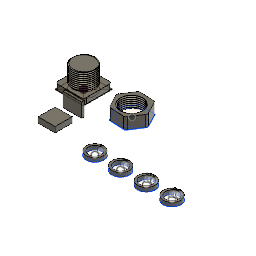
FineABSThreadTest (Autodesk Fusion 360 design; units mm, degrees)
Autodesk Fusion 360 part; units mm, degrees
sketch "Sketch1" plane through (0, 0, 0) normal (0, 1, 0) x (1, 0, 0)
  line L0 (25, 25) -> (-25, 25)
  line L1 (-25, 25) -> (-25, -25)
  line L2 (-25, -25) -> (25, -25)
  line L3 (25, -25) -> (25, 25)
  line L4 (25, 25) -> (-25, -25) construction
  line L5 (-25, 25) -> (25, -25) construction
  circle A0 centre (0, 0) radius 20
  circle A1 centre (85, 0) radius 20
  line L6 (100.5694, 24.4662) -> (71.5964, 25.7166)
  line L7 (71.5964, 25.7166) -> (56.027, 1.2504)
  line L8 (56.027, 1.2504) -> (69.4306, -24.4662)
  line L9 (69.4306, -24.4662) -> (98.4036, -25.7166)
  line L10 (98.4036, -25.7166) -> (113.973, -1.2504)
  line L11 (113.973, -1.2504) -> (100.5694, 24.4662)
  dimension "d1" = 50
  dimension "d2" = 50
  dimension "d3" = 40
  dimension "d4" = 40
  dimension "d5" = 29
  measures "d3" diameter of A0
  measures "d4" diameter of A1
extrude "Extrude1" add sketch "Sketch1" along normal blind 20 contours L6 L7 L8 L9 L10 L11 makes body 1
extrude "Extrude2" add sketch "Sketch1" along normal blind 10 separate body contours L0 L1 L2 L3 | A0 makes body 2
extrude "Extrude3" add sketch "Sketch1" along normal blind 40 contours A0 bodies 2
thread "Thread1" "ISO Metric profile 40.0 M40x3 6g" major diameter 39.7645 minor diameter 36.3299 pitch 3 angle 60 modelled right hand crest width 0.375 on face at (19.9006, 20, -1.9914) crest through (19.8822, 9.8125, 0) on bodies 2
thread "Thread2" "ISO Metric profile 40.0 M40x3 6H" major diameter 40.349 minor diameter 37.0024 pitch 3 angle 60 modelled right hand crest width 0.375 on face at (104.9751, 13.3333, 0.9969) crest through (103.5012, -1.6875, 0) on bodies 1
fillet "Fillet1" radius 5 4 edges at (25, 5, 25) (-25, 5, 25) (-25, 5, -25) (25, 5, -25) on bodies 2
fillet "Fillet2" radius 5 6 edges at (100.5694, 10, -24.4662) (71.5964, 10, -25.7166) (56.027, 10, -1.2504) (69.4306, 10, 24.4662) (98.4036, 10, 25.7166) (113.973, 10, 1.2504) on bodies 1
sketch "Sketch2" plane through (0, 0, 0) normal (0, 1, 0) x (1, 0, 0)
  line L0 (9.9496, -41.7476) -> (42.9679, -41.7476)
  line L1 (42.9679, -41.7476) -> (42.9679, -46.0778)
  line L2 (42.9679, -46.0778) -> (9.9496, -46.0778)
  line L3 (9.9496, -46.0778) -> (9.9496, -41.7476)
extrude "Extrude4" add sketch "Sketch2" along normal blind 25 separate body makes body 3
sketch "Sketch3" plane through (0, 0, 0) normal (0, 1, 0) x (1, 0, 0)
  line L0 (11.6785, -61.4289) -> (41.6785, -61.4289)
  line L1 (41.6785, -61.4289) -> (41.6785, -91.4289)
  line L2 (41.6785, -91.4289) -> (11.6785, -91.4289)
  line L3 (11.6785, -91.4289) -> (11.6785, -61.4289)
  dimension "d16" = 30
  dimension "d17" = 30
  measures "d16" distance of origin
extrude "Extrude5" add sketch "Sketch3" along normal blind 10 separate body makes body 4
sketch "Sketch4" plane through (0, 0, 0) normal (0, 0, 1) x (1, 0, 0)
sketch "Sketch5" plane through (0, 0, 0) normal (0, 1, 0) x (1, 0, 0)
  circle A0 centre (155, -90) radius 11.25
  circle A1 centre (155, -90) radius 15.25
  circle A2 centre (200, -90) radius 11.3
  circle A3 centre (200, -90) radius 15.3
  circle A4 centre (245, -90) radius 11.35
  circle A5 centre (245, -90) radius 15.35
  circle A6 centre (110, -90) radius 11.2
  circle A7 centre (110, -90) radius 15.2
  circle A8 centre (108, -77) radius 1
  circle A9 centre (149, -78) radius 1.4142
  circle A10 centre (153, -77) radius 1.4142
  circle A11 centre (191, -80) radius 1.4142
  circle A12 centre (195, -77) radius 1
  circle A13 centre (201, -77) radius 1
  circle A14 centre (236, -81) radius 1.4142
  circle A15 centre (238, -78) radius 1.4142
  circle A16 centre (241.5663, -78) radius 1.09
  circle A17 centre (244, -76) radius 1
  dimension "d20" = 22.5
  dimension "d21" = 4
  dimension "d22" = 22.6
  dimension "d23" = 4
  dimension "d24" = 22.7
  dimension "d25" = 4
  dimension "d26" = 22.4
  dimension "d27" = 4
  measures "d20" diameter of A0
  measures "d22" diameter of A2
  measures "d24" diameter of A4
  measures "d26" diameter of A6
extrude "Extrude6" add sketch "Sketch5" along normal blind 7 separate body contours A1 | A3 | A4 A14 | A5 | A7 | A8 | A9 | A10 | A11 | A12 | A13 | A15 | A16 | A17 picked at (235.5943, -80.7285) makes body 5 at (170.231, 2.3333, 90.7601) makes body 6 at (215.224, 4.6667, 91.5234) makes body 7 at (125.1245, 4.6667, 91.5134) makes body 8 at (260.2737, 4.6667, 91.5284)
extrude "Extrude7" add sketch "Sketch5" along normal blind 8.049 contours A4 A14 | A8 | A9 | A10 | A11 | A12 | A13 | A15 | A16 | A17 picked at (235.5943, -80.7285) bodies 5 6 7 8
